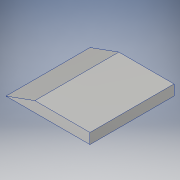
# Autodesk Inventor part: BallGuideHardstop
Saved by Autodesk Inventor 2018.3 (Build 223284000, 284)
## iProperties
Created: 2020-02-15
Part Number: BallGuideHardstop
Material: Aluminum 6061
Document SubType Name: Modeling
Designer: 22oktynich
Density: 2.7 g/cm^3
Appearance: Aluminum - Flat
Author: 22oktynich
Autodesk Inventor part; units mm, degrees
ref_plane "YZ Plane" through (0, 0, 0) normal (1, 0, 0) x (0, 1, 0)
ref_plane "XZ Plane" through (0, 0, 0) normal (0, 1, 0) x (-1, 0, 0)
ref_plane "XY Plane" through (0, 0, 0) normal (0, 0, 1) x (1, 0, 0)
sketch "Sketch1" plane through (0, 0, 0) normal (0, 0, 1) x (1, 0, 0)
  line L0 (0, 0) -> (-25.4, 0)
  line L1 (-16.6768, 3.175) -> (0, 3.175)
  line L2 (0, 3.175) -> (0, 0)
  line L3 (-25.4, 0) -> (-16.6768, 3.175)
  dimension "d0" = 20
  dimension "d2" = 3.175
  dimension "d3" = 25.4
  constraints: 8 end point, 1 horizontal, 1 parallel, 1 vertical
  measures "d0" angle of L0 L3
  measures "d2" distance of L1.end L0.start
  measures "d3" distance from line of L2 L0.end
extrude "Extrusion1" add sketch "Sketch1" along normal blind 25.4
body "Solid1"
